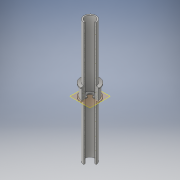
# Autodesk Inventor part: Middle beam
Saved by Autodesk Inventor 2016 SP1 (Build 200210100, 210)
## iProperties
Created: 2016-02-19
Part Number: Middle beam
Material: Generic
Document SubType Name: Modeling
Designer: Tore Den Store
Density: 1 g/cm^3
Appearance: Default
Author: Tore Den Store
Autodesk Inventor part; units mm, degrees
ref_plane "YZ Plane" through (0, 0, 0) normal (1, 0, 0) x (0, 1, 0)
ref_plane "XZ Plane" through (0, 0, 0) normal (0, 1, 0) x (-1, 0, 0)
ref_plane "XY Plane" through (0, 0, 0) normal (0, 0, 1) x (1, 0, 0)
sketch "Sketch1" plane through (0, 0, 0) normal (0, 0, 1) x (1, 0, 0)
  circle A0 centre (0, 0) radius 130
  dimension "d0" = 260
  constraints: 1 centre point, 1 coincident
  measures "d0" diameter of A0
extrude "Extrusion1" add sketch "Sketch1" along normal blind 180
sketch "Sketch2" plane through (0, 0, 180) normal (0, 0, 1) x (1, 0, 0)
  circle A0 centre (0, 0) radius 150
  dimension "d3" = 300
  constraints: 1 centre point, 1 coincident
  measures "d3" diameter of A0
extrude "Extrusion2" add sketch "Sketch2" along normal blind 15
sketch "Sketch3" plane through (0, 0, 195) normal (0, 0, 1) x (1, 0, 0)
  circle A0 centre (0, 0) radius 100
  dimension "d6" = 200
  constraints: 1 centre point, 1 coincident
  measures "d6" diameter of A0
extrude "Extrusion3" add sketch "Sketch3" along normal blind 900
ref_plane "Work Plane1" through (0, 0, 90) normal (0, 0, -1) x (-1, 0, 0)
mirror "Mirror1" about plane through (0, 0, 90) normal (0, 0, -1) of "Extrusion2", "Extrusion3"
hole "Hole1" at (0, 0, 1095) direction (0, 0, -1) diameter 160 end through all
ref_plane "Work Plane2" through (0, 0, 0) normal (0, 0, 1) x (1, 0, 0)
sketch "Sketch4" plane through (0, 0, 0) normal (0, 0, 1) x (1, 0, 0)
  circle A0 centre (0, 0) radius 80 projected
  circle A1 centre (0, 0) radius 40
  dimension "d19" = 40
  constraints: 1 centre point
  measures "d19" radial gap between concentric circles of A0 A1
extrude "Extrusion5" add sketch "Sketch4" along normal blind 15 separate body
body "Solid1"
body "Solid2"
